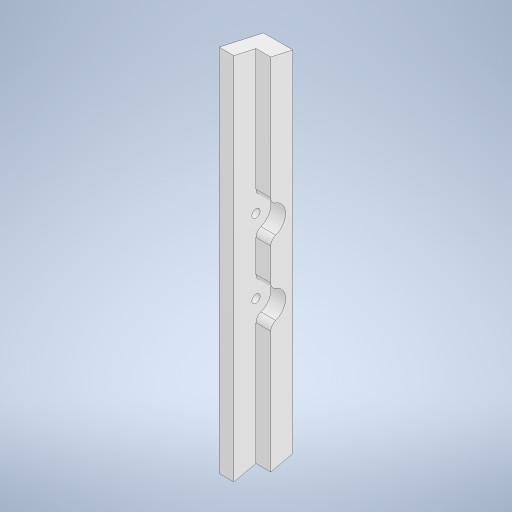
# Autodesk Inventor part: Legs
Saved by Autodesk Inventor 2023.1 (Build 271208000, 208)
## iProperties
Created: 2022-05-26
Part Number: Legs
Material: UHMW, White
Document SubType Name: Modeling
Designer: Nathan Cai
Mass: 23.25 g
Surface Area: 109.983 cm^2
Volume: 24.734 cm^3
Density: 0.94 g/cm^3
Appearance: Smooth - White
Author: Nathan Cai
Autodesk Inventor part; units mm, degrees
ref_plane "YZ Plane" through (0, 0, 0) normal (1, 0, 0) x (0, 1, 0)
ref_plane "XZ Plane" through (0, 0, 0) normal (0, 1, 0) x (-1, 0, 0)
ref_plane "XY Plane" through (0, 0, 0) normal (0, 0, 1) x (1, 0, 0)
sketch "Sketch1" plane through (0, 0, 0) normal (1, 0, 0) x (0, 1, 0)
  line L0 (79.375, 0) -> (79.375, 19.05)
  line L1 (79.375, 19.05) -> (0, 19.05)
  line L2 (0, 19.05) -> (0, 0) construction
  line L3 (0, 0) -> (79.375, 0)
  line L4 (-79.375, 0) -> (-79.375, 19.05)
  line L5 (-79.375, 19.05) -> (0, 19.05)
  line L6 (0, 0) -> (-79.375, 0)
  line L7 (-6.35, 9.525) -> (6.35, 9.525) construction
  circle A0 centre (15.875, 9.525) radius 1.7526
  circle A1 centre (-15.875, 9.525) radius 1.7526
  point P0 (-31.75, 0)
  point P1 (0, 9.525)
  dimension "d0" = 79.375
  dimension "d1" = 19.05
  dimension "d16" = 9.525
  dimension "d17" = 3.5052
  dimension "Leg_Holes" = 15.875
  dimension "d19" = 9.525
  dimension "d21" = 9.525
  constraints: 18 end point, 3 symmetric about line, 2 centre point, 2 midpoint, 2 parallel, 2 perpendicular, 2 point on line, 1 horizontal, 1 other
  measures "d0" distance of L1.end L0.end
  measures "d1" distance of L0.end L0.start
  measures "d16" distance between parallel lines of L5 L7
  measures "d17" diameter of A0
  measures "Leg_Holes" distance from line of L2 A0.centre
  measures "d19" distance from line of L1 A0.centre
  measures "d21" distance of A0.centre L7.end
extrude "Extrusion1" add sketch "Sketch1" along normal blind 6.35
chamfer "Chamfer1" distance 19.05 angle 12.5 1 edges at (3.175, 79.375, 0) measured on face at (3.175, 79.375, 0.5)
chamfer "Chamfer2" distance 19.05 angle 12.5 1 edges at (3.175, -79.375, 0) measured on face at (3.175, -79.375, 0.5)
sketch "Sketch3" plane through (6.35, 0, 0) normal (1, 0, 0) x (0, 0, -1)
  circle A0 centre (-9.525, 15.875) radius 1.7526 projected
  circle A1 centre (-9.525, 15.875) radius 6.35
  circle A2 centre (-9.525, -15.875) radius 1.7526 projected
  circle A3 centre (-9.525, -15.875) radius 6.35
  line L0 (0, 75.1517) -> (-19.05, 79.375) projected
  line L1 (-9.525, 77.2634) -> (0, 77.2634)
  line L2 (0, 77.2634) -> (0, -77.2634)
  line L3 (0, -77.2634) -> (-9.525, -77.2634)
  line L4 (-9.525, -77.2634) -> (-9.525, 77.2634)
  line L5 (0, -75.1517) -> (-19.05, -79.375) projected
  line L6 (0, -75.1517) -> (0, 75.1517) projected
  point P0 (0, 0)
  point P1 (-9.525, 22.225)
  point P2 (-9.525, 9.525)
  point P3 (-9.525, -9.525)
  point P4 (-9.525, -22.225)
  dimension "d28" = 12.7
  dimension "d29" = 12.7
  constraints: 8 end point, 3 midpoint, 2 centre point, 2 coincident, 2 parallel, 1 horizontal, 1 perpendicular, 1 point on line
  measures "d28" diameter of A1
  measures "d29" diameter of A3
extrude "Extrusion3" add sketch "Sketch3" along normal blind 6.35 contours L4 L0 L2 L5 A3 A1
fillet "Fillet4" radius 3.175 4 edges at (9.525, -22.225, 9.525) (9.525, -9.525, 9.525) (9.525, 9.525, 9.525) (9.525, 22.225, 9.525)
equation "\"d16\" = 0.5 * d1"
equation "\"Leg_Holes\" = Leg_Mounts"
equation "\"d19\" = d16"
equation "\"Leg_Mounts\" = 15.875"
body "Solid1"
